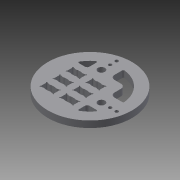
# Autodesk Inventor part: Segment_Med
Saved by Autodesk Inventor 2014 SP1 (Build 180222100, 222)
## iProperties
Created: 2012-09-02
Part Number: Segment_Med
Material: Generic
Document SubType Name: Modeling
Designer: ErikEnvy
Density: 1 g/cm^3
Appearance: Default
Author: ErikEnvy
Autodesk Inventor part; units mm, degrees
ref_plane "YZ Plane" through (0, 0, 0) normal (1, 0, 0) x (0, 1, 0)
ref_plane "XZ Plane" through (0, 0, 0) normal (0, 1, 0) x (-1, 0, 0)
ref_plane "XY Plane" through (0, 0, 0) normal (0, 0, 1) x (1, 0, 0)
sketch "Sketch1" plane through (0, 0, 0) normal (0, 0, 1) x (1, 0, 0)
  circle A0 centre (0, 13) radius 1.6
  circle A1 centre (13, 0) radius 1.6
  circle A2 centre (0, 17) radius 0.75
  circle A3 centre (17, 0) radius 0.75
  circle A4 centre (20, 0) radius 0.75
  circle A5 centre (0, 20) radius 0.75
  arc A6 (-7.25, 7.5) -> (-7.5, 7.25) centre (-7.5, 7.5) ccw
  arc A7 (-6.75, 7.5) -> (-5.25, 7.5) centre (-6, 8.8062) ccw
  arc A8 (-1.5, 7.25) -> (-1.75, 7.5) centre (-1.5, 7.5) ccw
  arc A9 (-3.75, 7.5) -> (-2.25, 7.5) centre (-3, 8.8062) ccw
  arc A10 (-7.5, 4.75) -> (-7.25, 4.5) centre (-7.5, 4.5) ccw
  arc A11 (-5.25, 4.5) -> (-6.75, 4.5) centre (-6, 3.1938) ccw
  arc A12 (-2.25, 4.5) -> (-3.75, 4.5) centre (-3, 3.1938) ccw
  arc A13 (-1.75, 4.5) -> (-1.5, 4.75) centre (-1.5, 4.5) ccw
  line L0 (-1.5, 7.25) -> (-1.5, 4.75)
  line L1 (-1.75, 4.5) -> (-2.25, 4.5)
  line L2 (-2.25, 7.5) -> (-1.75, 7.5)
  line L3 (-3.75, 7.5) -> (-5.25, 7.5)
  line L4 (-5.25, 4.5) -> (-3.75, 4.5)
  line L5 (-7.25, 7.5) -> (-6.75, 7.5)
  line L6 (-7.5, 7.25) -> (-7.5, 4.75)
  line L7 (-6.75, 4.5) -> (-7.25, 4.5)
  arc A14 (1.75, 7.5) -> (1.5, 7.25) centre (1.5, 7.5) ccw
  arc A15 (2.25, 7.5) -> (3.75, 7.5) centre (3, 8.8062) ccw
  arc A16 (5.25, 7.5) -> (6.75, 7.5) centre (6, 8.8062) ccw
  arc A17 (7.5, 7.25) -> (7.25, 7.5) centre (7.5, 7.5) ccw
  arc A18 (6.75, 4.5) -> (5.25, 4.5) centre (6, 3.1938) ccw
  arc A19 (7.25, 4.5) -> (7.5, 4.75) centre (7.5, 4.5) ccw
  arc A20 (3.75, 4.5) -> (2.25, 4.5) centre (3, 3.1938) ccw
  arc A21 (1.5, 4.75) -> (1.75, 4.5) centre (1.5, 4.5) ccw
  line L8 (7.5, 7.25) -> (7.5, 4.75)
  line L9 (7.25, 4.5) -> (6.75, 4.5)
  line L10 (6.75, 7.5) -> (7.25, 7.5)
  line L11 (5.25, 7.5) -> (3.75, 7.5)
  line L12 (3.75, 4.5) -> (5.25, 4.5)
  line L13 (1.75, 7.5) -> (2.25, 7.5)
  line L14 (1.5, 7.25) -> (1.5, 4.75)
  line L15 (2.25, 4.5) -> (1.75, 4.5)
  arc A22 (-7.25, 1.5) -> (-7.5, 1.25) centre (-7.5, 1.5) ccw
  arc A23 (-6.75, 1.5) -> (-5.25, 1.5) centre (-6, 2.8062) ccw
  arc A24 (-3.75, 1.5) -> (-2.25, 1.5) centre (-3, 2.8062) ccw
  arc A25 (-1.5, 1.25) -> (-1.75, 1.5) centre (-1.5, 1.5) ccw
  arc A26 (-2.25, -1.5) -> (-3.75, -1.5) centre (-3, -2.8062) ccw
  arc A27 (-1.75, -1.5) -> (-1.5, -1.25) centre (-1.5, -1.5) ccw
  arc A28 (-5.25, -1.5) -> (-6.75, -1.5) centre (-6, -2.8062) ccw
  arc A29 (-7.5, -1.25) -> (-7.25, -1.5) centre (-7.5, -1.5) ccw
  line L16 (-1.5, 1.25) -> (-1.5, -1.25)
  line L17 (-1.75, -1.5) -> (-2.25, -1.5)
  line L18 (-2.25, 1.5) -> (-1.75, 1.5)
  line L19 (-3.75, 1.5) -> (-5.25, 1.5)
  line L20 (-5.25, -1.5) -> (-3.75, -1.5)
  line L21 (-7.25, 1.5) -> (-6.75, 1.5)
  line L22 (-7.5, 1.25) -> (-7.5, -1.25)
  line L23 (-6.75, -1.5) -> (-7.25, -1.5)
  arc A30 (1.75, 1.5) -> (1.5, 1.25) centre (1.5, 1.5) ccw
  arc A31 (2.25, 1.5) -> (3.75, 1.5) centre (3, 2.8062) ccw
  arc A32 (5.25, 1.5) -> (6.75, 1.5) centre (6, 2.8062) ccw
  arc A33 (7.5, 1.25) -> (7.25, 1.5) centre (7.5, 1.5) ccw
  arc A34 (6.75, -1.5) -> (5.25, -1.5) centre (6, -2.8062) ccw
  arc A35 (7.25, -1.5) -> (7.5, -1.25) centre (7.5, -1.5) ccw
  arc A36 (3.75, -1.5) -> (2.25, -1.5) centre (3, -2.8062) ccw
  arc A37 (1.5, -1.25) -> (1.75, -1.5) centre (1.5, -1.5) ccw
  line L24 (7.5, 1.25) -> (7.5, -1.25)
  line L25 (7.25, -1.5) -> (6.75, -1.5)
  line L26 (6.75, 1.5) -> (7.25, 1.5)
  line L27 (5.25, 1.5) -> (3.75, 1.5)
  line L28 (3.75, -1.5) -> (5.25, -1.5)
  line L29 (1.75, 1.5) -> (2.25, 1.5)
  line L30 (1.5, 1.25) -> (1.5, -1.25)
  line L31 (2.25, -1.5) -> (1.75, -1.5)
  arc A38 (-7.25, -4.5) -> (-7.5, -4.75) centre (-7.5, -4.5) ccw
  arc A39 (-6.75, -4.5) -> (-5.25, -4.5) centre (-6, -3.1938) ccw
  arc A40 (-3.75, -4.5) -> (-2.25, -4.5) centre (-3, -3.1938) ccw
  arc A41 (-1.5, -4.75) -> (-1.75, -4.5) centre (-1.5, -4.5) ccw
  arc A42 (-2.25, -7.5) -> (-3.75, -7.5) centre (-3, -8.8062) ccw
  arc A43 (-1.75, -7.5) -> (-1.5, -7.25) centre (-1.5, -7.5) ccw
  arc A44 (-5.25, -7.5) -> (-6.75, -7.5) centre (-6, -8.8062) ccw
  arc A45 (-7.5, -7.25) -> (-7.25, -7.5) centre (-7.5, -7.5) ccw
  line L32 (-1.5, -4.75) -> (-1.5, -7.25)
  line L33 (-1.75, -7.5) -> (-2.25, -7.5)
  line L34 (-2.25, -4.5) -> (-1.75, -4.5)
  line L35 (-3.75, -4.5) -> (-5.25, -4.5)
  line L36 (-5.25, -7.5) -> (-3.75, -7.5)
  line L37 (-7.25, -4.5) -> (-6.75, -4.5)
  line L38 (-7.5, -4.75) -> (-7.5, -7.25)
  line L39 (-6.75, -7.5) -> (-7.25, -7.5)
  arc A46 (1.75, -4.5) -> (1.5, -4.75) centre (1.5, -4.5) ccw
  arc A47 (2.25, -4.5) -> (3.75, -4.5) centre (3, -3.1938) ccw
  arc A48 (5.25, -4.5) -> (6.75, -4.5) centre (6, -3.1938) ccw
  arc A49 (7.5, -4.75) -> (7.25, -4.5) centre (7.5, -4.5) ccw
  arc A50 (6.75, -7.5) -> (5.25, -7.5) centre (6, -8.8062) ccw
  arc A51 (7.25, -7.5) -> (7.5, -7.25) centre (7.5, -7.5) ccw
  arc A52 (3.75, -7.5) -> (2.25, -7.5) centre (3, -8.8062) ccw
  arc A53 (1.5, -7.25) -> (1.75, -7.5) centre (1.5, -7.5) ccw
  line L40 (7.5, -4.75) -> (7.5, -7.25)
  line L41 (7.25, -7.5) -> (6.75, -7.5)
  line L42 (6.75, -4.5) -> (7.25, -4.5)
  line L43 (5.25, -4.5) -> (3.75, -4.5)
  line L44 (3.75, -7.5) -> (5.25, -7.5)
  line L45 (1.75, -4.5) -> (2.25, -4.5)
  line L46 (1.5, -4.75) -> (1.5, -7.25)
  line L47 (2.25, -7.5) -> (1.75, -7.5)
  circle A54 centre (3.8891, 3.8891) radius 19.25
  line L48 (5, 14) -> (5, 17.5444)
  line L49 (17.5444, 5) -> (14, 5)
  line L50 (12, 7) -> (12, 10)
  arc A55 (18.041, 5.5586) -> (5.5586, 18.041) centre (3.8891, 3.8891) ccw
  line L51 (10, 12) -> (7, 12)
  line L52 (11.5, -4) -> (14.7834, -4)
  line L53 (10.5, -7.8794) -> (10.5, -5)
  line L54 (-4, 14.7834) -> (-4, 11.5)
  line L55 (-5, 10.5) -> (-7.8794, 10.5)
  arc A56 (11.2586, -8.3074) -> (15.1795, -4.8051) centre (3.8891, 3.8891) ccw
  arc A57 (-4.8051, 15.1795) -> (-8.3074, 11.2586) centre (3.8891, 3.8891) ccw
  arc A58 (12, 10) -> (10, 12) centre (10, 10) ccw
  arc A59 (12, 7) -> (14, 5) centre (14, 7) ccw
  arc A60 (5, 14) -> (7, 12) centre (7, 14) ccw
  arc A61 (-5, 10.5) -> (-4, 11.5) centre (-5, 11.5) ccw
  arc A62 (11.5, -4) -> (10.5, -5) centre (11.5, -5) ccw
  arc A63 (-8.3074, 11.2586) -> (-7.8794, 10.5) centre (-7.8794, 11) ccw
  arc A64 (-4, 14.7834) -> (-4.8051, 15.1795) centre (-4.5, 14.7834) ccw
  arc A65 (5.5586, 18.041) -> (5, 17.5444) centre (5.5, 17.5444) ccw
  arc A66 (17.5444, 5) -> (18.041, 5.5586) centre (17.5444, 5.5) ccw
  arc A67 (15.1795, -4.8051) -> (14.7834, -4) centre (14.7834, -4.5) ccw
  arc A68 (10.5, -7.8794) -> (11.2586, -8.3074) centre (11, -7.8794) ccw
  point P0 (5, 18.0957)
  point P1 (18.0957, 5)
  point P2 (15.756, -4)
  point P3 (10.5, -8.7346)
  point P4 (-4, 15.756)
  point P5 (-8.7346, 10.5)
  constraints: 130 point on circle, 112 end point, 69 centre point, 22 tangent, 8 equal radius, 6 point on line, 3 parallel, 3 perpendicular, 2 horizontal, 1 coincident, 1 collinear, 1 vertical, 2 other
extrude "Extrusion1" add sketch "Sketch1" along normal blind 3
body "Solid1"
